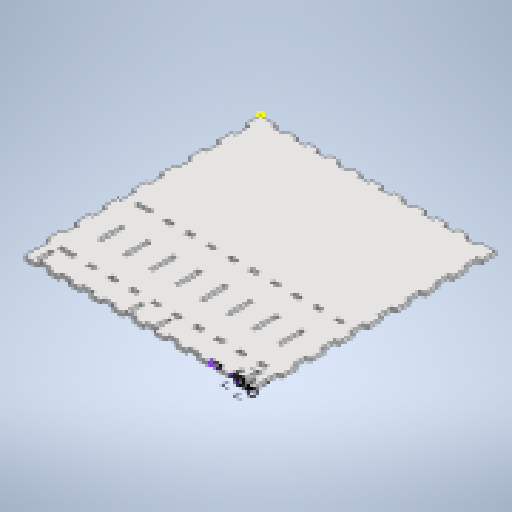
# Autodesk Inventor part: Bottom
Saved by Autodesk Inventor 2023 (Build 270158000, 158)
## iProperties
Created: 2023-08-30
Part Number: Bottom
Material: Generic
Document SubType Name: Modeling
Designer: Nathann
Density: 1 g/cm^3
Appearance: Default
Author: Nathann
Autodesk Inventor part; units mm, degrees
ref_plane "YZ Plane" through (0, 0, 0) normal (1, 0, 0) x (0, 1, 0)
ref_plane "XZ Plane" through (0, 0, 0) normal (0, 1, 0) x (-1, 0, 0)
ref_plane "XY Plane" through (0, 0, 0) normal (0, 0, 1) x (1, 0, 0)
sketch "Sketch1" plane through (0, 0, 0) normal (0, 1, 0) x (-1, 0, 0)
  line L0 (0, 0) -> (-330, 0)
  line L1 (-330, 0) -> (-330, 330)
  line L2 (-330, 330) -> (0, 330)
  line L3 (0, 330) -> (0, 0)
  dimension "d0" = 330
  dimension "d1" = 330
  constraints: 8 end point, 2 parallel, 1 horizontal, 1 perpendicular
  measures "d0" distance of L2.end L0.start
  measures "d1" distance of L1.end L2.end
extrude "Extrusion1" add sketch "Sketch1" along normal blind 5
sketch "Sketch4" plane through (0, 0, 0) normal (0, -1, 0) x (1, 0, 0)
  line L0 (325, 325) -> (307.5, 325) projected
  line L1 (325, 330) -> (325, 300) projected
  line L2 (307.5, 325) -> (307.5, 330) projected
  line L3 (0, 330) -> (330, 330) projected
  line L4 (297.5, 325) -> (297.5, 330)
  line L5 (277.5, 325) -> (277.5, 330) projected
  line L6 (292.5, 325) -> (277.5, 325) projected
  line L7 (292.5, 330) -> (292.5, 325) projected
  line L8 (262.5, 330) -> (262.5, 325) projected
  line L9 (262.5, 325) -> (247.5, 325) projected
  line L10 (247.5, 325) -> (247.5, 330) projected
  line L11 (232.5, 330) -> (232.5, 325) projected
  line L12 (232.5, 325) -> (217.5, 325) projected
  line L13 (217.5, 325) -> (217.5, 330) projected
  line L14 (202.5, 330) -> (202.5, 325) projected
  line L15 (202.5, 325) -> (187.5, 325) projected
  line L16 (187.5, 325) -> (187.5, 330) projected
  line L17 (172.5, 330) -> (172.5, 325) projected
  line L18 (172.5, 325) -> (157.5, 325) projected
  line L19 (157.5, 325) -> (157.5, 330) projected
  line L20 (142.5, 325) -> (127.5, 325) projected
  line L21 (142.5, 330) -> (142.5, 325) projected
  line L22 (127.5, 325) -> (127.5, 330) projected
  line L23 (112.5, 330) -> (112.5, 325) projected
  line L24 (112.5, 325) -> (97.5, 325) projected
  line L25 (97.5, 325) -> (97.5, 330) projected
  line L26 (82.5, 325) -> (67.5, 325) projected
  line L27 (82.5, 330) -> (82.5, 325) projected
  line L28 (67.5, 325) -> (67.5, 330) projected
  line L29 (52.5, 325) -> (37.5, 325) projected
  line L30 (52.5, 330) -> (52.5, 325) projected
  line L31 (37.5, 325) -> (37.5, 330) projected
  line L32 (22.5, 325) -> (5, 325) projected
  line L33 (22.5, 330) -> (22.5, 325) projected
  line L34 (5, 330) -> (5, 300) projected
  line L35 (292.5, 325) -> (307.5, 325) projected
  line L36 (262.5, 325) -> (277.5, 325) projected
  line L37 (232.5, 325) -> (247.5, 325) projected
  line L38 (202.5, 325) -> (217.5, 325) projected
  line L39 (172.5, 325) -> (187.5, 325) projected
  line L40 (142.5, 325) -> (157.5, 325) projected
  line L41 (112.5, 325) -> (127.5, 325) projected
  line L42 (82.5, 325) -> (97.5, 325) projected
  line L43 (52.5, 325) -> (67.5, 325) projected
  line L44 (22.5, 325) -> (37.5, 325) projected
  line L45 (0, 300) -> (5, 300) projected
  line L46 (5, 300) -> (5, 280) projected
  line L47 (0, 330) -> (0, 300) projected
  line L48 (0, 0) -> (0, 330) projected
  line L49 (5, 280) -> (0, 280) projected
  line L50 (5, 280) -> (5, 260) projected
  line L51 (0, 260) -> (5, 260) projected
  line L52 (5, 260) -> (5, 240) projected
  line L53 (5, 240) -> (0, 240) projected
  line L54 (5, 240) -> (0, 240) projected
  line L55 (0, 240) -> (0, 220) projected
  line L56 (0, 220) -> (5, 220) projected
  line L57 (5, 240) -> (5, 220) projected
  line L58 (5, 220) -> (5, 200) projected
  line L59 (5, 200) -> (0, 200) projected
  line L60 (5, 200) -> (5, 180) projected
  line L61 (0, 180) -> (5, 180) projected
  line L62 (5, 180) -> (5, 160) projected
  line L63 (5, 160) -> (0, 160) projected
  line L64 (5, 160) -> (5, 140) projected
  line L65 (0, 140) -> (5, 140) projected
  line L66 (5, 140) -> (5, 120) projected
  line L67 (5, 120) -> (0, 120) projected
  line L68 (5, 120) -> (5, 100) projected
  line L69 (0, 100) -> (5, 100) projected
  line L70 (5, 100) -> (5, 80) projected
  line L71 (5, 80) -> (0, 80) projected
  line L72 (5, 80) -> (5, 60) projected
  line L73 (0, 60) -> (5, 60) projected
  line L74 (5, 60) -> (5, 40) projected
  line L75 (5, 40) -> (0, 40) projected
  line L76 (5, 40) -> (5, 20) projected
  line L77 (0, 20) -> (5, 20) projected
  line L78 (5, 20) -> (5, 0) projected
  line L79 (330, 0) -> (0, 0) projected
  line L80 (5, 5) -> (22.5, 5) projected
  line L81 (22.5, 5) -> (22.5, 0) projected
  line L82 (37.5, 0) -> (37.5, 5) projected
  line L83 (22.5, 5) -> (37.5, 5) projected
  line L84 (45, 0) -> (45, 5) projected
  line L85 (37.5, 5) -> (52.5, 5) projected
  line L86 (52.5, 5) -> (52.5, 0) projected
  line L87 (52.5, 5) -> (67.5, 5) projected
  line L88 (67.5, 0) -> (67.5, 5) projected
  line L89 (67.5, 5) -> (82.5, 5) projected
  line L90 (82.5, 5) -> (82.5, 0) projected
  line L91 (82.5, 5) -> (97.5, 5) projected
  line L92 (97.5, 0) -> (97.5, 5) projected
  line L93 (112.5, 5) -> (112.5, 0) projected
  line L94 (97.5, 5) -> (112.5, 5) projected
  line L95 (112.5, 5) -> (127.5, 5) projected
  line L96 (127.5, 0) -> (127.5, 5) projected
  line L97 (127.5, 5) -> (142.5, 5) projected
  line L98 (142.5, 5) -> (142.5, 0) projected
  line L99 (142.5, 5) -> (157.5, 5) projected
  line L100 (157.5, 0) -> (157.5, 5) projected
  line L101 (157.5, 5) -> (172.5, 5) projected
  line L102 (172.5, 5) -> (172.5, 0) projected
  line L103 (172.5, 5) -> (187.5, 5) projected
  line L104 (187.5, 0) -> (187.5, 5) projected
  line L105 (187.5, 5) -> (202.5, 5) projected
  line L106 (202.5, 5) -> (202.5, 0) projected
  line L107 (202.5, 5) -> (217.5, 5) projected
  line L108 (217.5, 0) -> (217.5, 5) projected
  line L109 (217.5, 5) -> (232.5, 5) projected
  line L110 (232.5, 5) -> (232.5, 0) projected
  line L111 (232.5, 5) -> (247.5, 5) projected
  line L112 (247.5, 0) -> (247.5, 5) projected
  line L113 (247.5, 5) -> (262.5, 5) projected
  line L114 (262.5, 5) -> (262.5, 0) projected
  line L115 (262.5, 5) -> (277.5, 5) projected
  line L116 (277.5, 0) -> (277.5, 5) projected
  line L117 (277.5, 5) -> (292.5, 5) projected
  line L118 (292.5, 5) -> (292.5, 0) projected
  line L119 (292.5, 5) -> (307.5, 5) projected
  line L120 (307.5, 0) -> (307.5, 5) projected
  line L121 (307.5, 5) -> (325, 5) projected
  line L122 (325, 0) -> (325, 5) projected
  line L123 (325, 5) -> (330, 5) projected
  line L124 (325, 0) -> (325, 20) projected
  line L125 (325, 40) -> (325, 20) projected
  line L126 (325, 20) -> (330, 20) projected
  line L127 (325, 20) -> (330, 20) projected
  line L128 (330, 40) -> (330, 20) projected
  line L129 (330, 40) -> (325, 40) projected
  line L130 (325, 40) -> (325, 20) projected
  line L131 (325, 40) -> (325, 60) projected
  line L132 (325, 60) -> (330, 60) projected
  line L133 (330, 80) -> (325, 80) projected
  line L134 (325, 80) -> (325, 60) projected
  line L135 (325, 80) -> (325, 100) projected
  line L136 (325, 100) -> (330, 100) projected
  line L137 (325, 120) -> (325, 100) projected
  line L138 (330, 120) -> (325, 120) projected
  line L139 (325, 120) -> (325, 140) projected
  line L140 (325, 140) -> (330, 140) projected
  line L141 (325, 140) -> (330, 140) projected
  line L142 (330, 160) -> (330, 140) projected
  line L143 (330, 160) -> (325, 160) projected
  line L144 (325, 160) -> (325, 140) projected
  line L145 (325, 160) -> (325, 180) projected
  line L146 (325, 180) -> (330, 180) projected
  line L147 (330, 330) -> (330, 0) projected
  line L148 (330, 200) -> (325, 200) projected
  line L149 (325, 200) -> (325, 180) projected
  line L150 (325, 180) -> (330, 180) projected
  line L151 (330, 200) -> (330, 180) projected
  line L152 (325, 220) -> (330, 220) projected
  line L153 (325, 200) -> (325, 220) projected
  line L154 (325, 240) -> (325, 220) projected
  line L155 (330, 240) -> (325, 240) projected
  line L156 (325, 240) -> (325, 260) projected
  line L157 (325, 260) -> (330, 260) projected
  line L158 (325, 280) -> (325, 260) projected
  line L159 (330, 280) -> (325, 280) projected
  line L160 (325, 280) -> (325, 300) projected
  line L161 (325, 300) -> (330, 300) projected
  line L162 (330, 325) -> (325, 325) projected
  line L163 (293.8889, 264) -> (288.8889, 264) projected
  line L164 (257.7778, 299) -> (257.7778, 264) projected
  line L165 (252.7778, 264) -> (252.7778, 299) projected
  line L166 (257.7778, 264) -> (252.7778, 264) projected
  line L167 (221.6667, 299) -> (221.6667, 264) projected
  line L168 (216.6667, 264) -> (216.6667, 299) projected
  line L169 (221.6667, 264) -> (216.6667, 264) projected
  line L170 (221.6667, 264) -> (221.6667, 231) projected
  line L171 (216.6667, 231) -> (216.6667, 264) projected
  line L172 (216.6667, 231) -> (221.6667, 231) projected
  line L173 (257.7778, 264) -> (257.7778, 231) projected
  line L174 (257.7778, 264) -> (252.7778, 264) projected
  line L175 (252.7778, 231) -> (252.7778, 264) projected
  line L176 (252.7778, 231) -> (257.7778, 231) projected
  line L177 (257.7778, 264) -> (257.7778, 231) projected
  line L178 (293.8889, 264) -> (288.8889, 264) projected
  line L179 (288.8889, 231) -> (288.8889, 264) projected
  line L180 (288.8889, 231) -> (293.8889, 231) projected
  line L181 (293.8889, 264) -> (293.8889, 231) projected
  line L182 (185.5556, 264) -> (180.5556, 264) projected
  line L183 (180.5556, 231) -> (180.5556, 264) projected
  line L184 (180.5556, 231) -> (185.5556, 231) projected
  line L185 (185.5556, 264) -> (185.5556, 231) projected
  line L186 (185.5556, 299) -> (185.5556, 264) projected
  line L187 (180.5556, 264) -> (180.5556, 299) projected
  line L188 (149.4444, 264) -> (144.4444, 264) projected
  line L189 (144.4444, 231) -> (144.4444, 264) projected
  line L190 (144.4444, 231) -> (149.4444, 231) projected
  line L191 (149.4444, 264) -> (149.4444, 231) projected
  line L192 (113.3333, 264) -> (108.3333, 264) projected
  line L193 (108.3333, 231) -> (108.3333, 264) projected
  line L194 (108.3333, 231) -> (113.3333, 231) projected
  line L195 (113.3333, 264) -> (113.3333, 231) projected
  line L196 (77.2222, 264) -> (72.2222, 264) projected
  line L197 (72.2222, 231) -> (72.2222, 264) projected
  line L198 (72.2222, 231) -> (77.2222, 231) projected
  line L199 (77.2222, 264) -> (77.2222, 231) projected
  line L200 (41.1111, 264) -> (36.1111, 264) projected
  line L201 (36.1111, 231) -> (36.1111, 264) projected
  line L202 (36.1111, 231) -> (41.1111, 231) projected
  line L203 (41.1111, 264) -> (41.1111, 231) projected
  line L204 (20, 196) -> (40, 196) projected
  line L205 (40, 191) -> (40, 196) projected
  line L206 (20, 196) -> (40, 196) projected
  line L207 (20, 196) -> (20, 191) projected
  line L208 (20, 191) -> (40, 191) projected
  line L209 (60, 196) -> (60, 191) projected
  line L210 (60, 191) -> (70, 191) projected
  line L211 (70, 191) -> (70, 196) projected
  line L212 (60, 196) -> (70, 196) projected
  line L213 (100, 191) -> (100, 196) projected
  line L214 (90, 196) -> (100, 196) projected
  line L215 (90, 196) -> (90, 191) projected
  line L216 (90, 191) -> (100, 191) projected
  line L217 (120, 196) -> (120, 191) projected
  line L218 (120, 191) -> (130, 191) projected
  line L219 (130, 191) -> (130, 196) projected
  line L220 (120, 196) -> (130, 196) projected
  line L221 (160, 191) -> (160, 196) projected
  line L222 (150, 196) -> (160, 196) projected
  line L223 (150, 196) -> (150, 191) projected
  line L224 (150, 191) -> (160, 191) projected
  line L225 (180, 196) -> (180, 191) projected
  line L226 (180, 191) -> (190, 191) projected
  line L227 (190, 191) -> (190, 196) projected
  line L228 (180, 196) -> (190, 196) projected
  line L229 (216.6667, 191) -> (216.6667, 196) projected
  line L230 (210, 196) -> (210, 191) projected
  line L231 (210, 191) -> (220, 191) projected
  line L232 (220, 191) -> (220, 196) projected
  line L233 (210, 196) -> (220, 196) projected
  line L234 (250, 191) -> (250, 196) projected
  line L235 (240, 196) -> (250, 196) projected
  line L236 (240, 196) -> (240, 191) projected
  line L237 (240, 191) -> (250, 191) projected
  line L238 (280, 191) -> (280, 196) projected
  line L239 (270, 196) -> (280, 196) projected
  line L240 (270, 196) -> (270, 191) projected
  line L241 (270, 191) -> (280, 191) projected
  line L242 (300, 196) -> (300, 191) projected
  line L243 (300, 191) -> (310, 191) projected
  line L244 (310, 191) -> (310, 196) projected
  line L245 (300, 196) -> (310, 196) projected
  line L246 (300, 191) -> (280, 191) projected
  point P0 (181.5, 325)
  constraints: 2 end point, 1 vertical, 7 other
extrude "Extrusion2" cut sketch "Sketch4" against normal blind 10 contours L162 L147 L161 L1 | L1 L3 L147 L162 | L35 L4 L3 L2 | L35 L7 L3 L4 | L159 L147 L157 L158 | L36 L8 L3 L5 | L155 L147 L152 L154 | L37 L11 L3 L10 | L148 L147 L146 L149 | L38 L14 L3 L13 | L143 L142 L140 L144 | L39 L17 L3 L16 | L138 L147 L136 L137 | L40 L21 L3 L19 | L133 L147 L132 L134 | L41 L23 L3 L22 | L129 L128 L126 L125 | L42 L27 L3 L25 | L120 L79 L118 L119 | L43 L30 L3 L28 | L116 L79 L114 L115 | L44 L33 L3 L31 | L112 L79 L110 L111 | L34 L45 L47 L3 | L108 L79 L106 L107 | L50 L51 L48 L49 | L104 L79 L102 L103 | L57 L56 L48 L53 | L100 L79 L98 L99 | L60 L61 L48 L59 | L96 L79 L93 L95 | L64 L65 L48 L63 | L92 L79 L90 L91 | L68 L69 L48 L67 | L88 L79 L86 L87 | L72 L73 L48 L71 | L76 L77 L48 L75 | L82 L79 L81 L83 | L181 L180 L179 L163 | L173 L176 L175 L166 | L170 L172 L171 L169 | L185 L184 L183 L182 | L191 L190 L189 L188 | L195 L194 L193 L192 | L199 L198 L197 L196 | L203 L202 L201 L200 | L204 L205 L208 L207 | L212 L211 L210 L209 | L216 L215 L214 L213 | L220 L219 L218 L217 | L224 L223 L222 L221 | L228 L227 L226 L225 | L231 L230 L233 L229 | L229 L233 L232 L231 | L237 L236 L235 L234 | L241 L240 L239 L238 | L242 L245 L244 L243
sketch "Sketch5" plane through (0, 0, 0) normal (0, -1, 0) x (1, 0, 0)
  line L0 (325, 304) -> (5, 304) projected
  line L1 (5, 299) -> (325, 299) projected
  line L2 (313.5, 304) -> (313.5, 325) projected
  line L3 (308.5, 304) -> (313.5, 304) projected
  line L4 (308.5, 325) -> (308.5, 304) projected
  line L5 (313.5, 325) -> (308.5, 325) projected
  line L6 (186.5, 304) -> (186.5, 325) projected
  line L7 (181.5, 304) -> (186.5, 304) projected
  line L8 (181.5, 325) -> (181.5, 304) projected
  line L9 (186.5, 325) -> (181.5, 325) projected
  line L10 (148.5, 304) -> (148.5, 325) projected
  line L11 (143.5, 304) -> (148.5, 304) projected
  line L12 (143.5, 325) -> (143.5, 304) projected
  line L13 (148.5, 325) -> (143.5, 325) projected
  line L14 (21.5, 304) -> (21.5, 325) projected
  line L15 (16.5, 304) -> (21.5, 304) projected
  line L16 (16.5, 325) -> (16.5, 304) projected
  line L17 (21.5, 325) -> (16.5, 325) projected
  line L18 (143.5, 310) -> (148.5, 310) projected
  line L19 (181.5, 310) -> (186.5, 310) projected
  line L20 (16.5, 310) -> (21.5, 310) projected
  line L21 (308.5, 310) -> (313.5, 310) projected
  line L22 (310, 299) -> (310, 304) projected
  line L23 (300, 304) -> (300, 299) projected
  line L24 (293.8889, 304) -> (293.8889, 299) projected
  line L25 (288.8889, 304) -> (288.8889, 299) projected
  line L26 (270, 304) -> (270, 299) projected
  line L27 (270, 299) -> (280, 299) projected
  line L28 (280, 299) -> (280, 304) projected
  line L29 (270, 304) -> (280, 304) projected
  line L30 (257.7778, 304) -> (257.7778, 299) projected
  line L31 (250, 299) -> (250, 304) projected
  line L32 (240, 304) -> (250, 304) projected
  line L33 (240, 304) -> (240, 299) projected
  line L34 (240, 299) -> (250, 299) projected
  line L35 (210, 304) -> (210, 299) projected
  line L36 (210, 299) -> (220, 299) projected
  line L37 (220, 299) -> (220, 304) projected
  line L38 (210, 304) -> (220, 304) projected
  line L39 (190, 299) -> (190, 304) projected
  line L40 (180, 304) -> (190, 304) projected
  line L41 (180, 304) -> (180, 299) projected
  line L42 (180, 299) -> (190, 299) projected
  line L43 (120, 304) -> (120, 299) projected
  line L44 (120, 299) -> (130, 299) projected
  line L45 (130, 299) -> (130, 304) projected
  line L46 (120, 304) -> (130, 304) projected
  line L47 (20, 304) -> (20, 299) projected
  line L48 (20, 299) -> (40, 299) projected
  line L49 (40, 299) -> (40, 304) projected
  line L50 (20, 304) -> (40, 304) projected
  line L51 (60, 304) -> (60, 299) projected
  line L52 (60, 299) -> (70, 299) projected
  line L53 (70, 299) -> (70, 304) projected
  line L54 (60, 304) -> (70, 304) projected
  line L55 (100, 299) -> (100, 304) projected
  line L56 (90, 304) -> (100, 304) projected
  line L57 (90, 304) -> (90, 299) projected
  line L58 (90, 299) -> (100, 299) projected
  line L59 (108.3333, 304) -> (108.3333, 299) projected
  line L60 (113.3333, 304) -> (113.3333, 299) projected
  line L61 (144.4444, 304) -> (144.4444, 299) projected
  line L62 (150, 304) -> (150, 299) projected
  line L63 (149.4444, 304) -> (149.4444, 299) projected
  line L64 (160, 299) -> (160, 304) projected
  point P0 (0, 0)
  constraints: 2 other
extrude "Extrusion3" cut sketch "Sketch5" against normal blind 10 contours L22 L1 L23 L0 | L21 L4 L5 L2 | L28 L1 L26 L0 | L31 L1 L33 L0 | L37 L1 L35 L0 | L39 L1 L41 L0 | L19 L8 L9 L6 | L1 L62 L0 L64 | L1 L43 L0 L45 | L18 L12 L13 L10 | L1 L57 L0 L55 | L1 L51 L0 L53 | L1 L47 L0 L49 | L20 L16 L17 L14
sketch "Sketch6" plane through (0, 0, 0) normal (0, -1, 0) x (1, 0, 0)
  line L0 (325, 300) -> (325, 330) projected
  line L1 (325, 330) -> (307.5, 330)
  line L2 (307.5, 330) -> (307.5, 336)
  line L3 (307.5, 336) -> (325, 336)
  line L4 (325, 336) -> (325, 330)
  line L5 (307.5, 325) -> (292.5, 325) projected
  line L6 (307.5, 325) -> (292.5, 325)
  line L7 (292.5, 325) -> (292.5, 331)
  line L8 (292.5, 331) -> (307.5, 331)
  line L9 (307.5, 331) -> (307.5, 325)
  line L10 (277.5, 330) -> (292.5, 330) projected
  line L11 (292.5, 330) -> (277.5, 330)
  line L12 (277.5, 330) -> (277.5, 336)
  line L13 (277.5, 336) -> (292.5, 336)
  line L14 (292.5, 336) -> (292.5, 330)
  line L15 (277.5, 330) -> (277.5, 325) projected
  line L16 (277.5, 325) -> (262.5, 325)
  line L17 (262.5, 325) -> (262.5, 331)
  line L18 (262.5, 331) -> (277.5, 331)
  line L19 (277.5, 331) -> (277.5, 325)
  line L20 (262.5, 325) -> (262.5, 330) projected
  line L21 (262.5, 330) -> (247.5, 330)
  line L22 (247.5, 330) -> (247.5, 336)
  line L23 (247.5, 336) -> (262.5, 336)
  line L24 (262.5, 336) -> (262.5, 330)
  line L25 (247.5, 330) -> (247.5, 325) projected
  line L26 (247.5, 325) -> (232.5, 325)
  line L27 (232.5, 325) -> (232.5, 331)
  line L28 (232.5, 331) -> (247.5, 331)
  line L29 (247.5, 331) -> (247.5, 325)
  line L30 (217.5, 330) -> (232.5, 330) projected
  line L31 (232.5, 330) -> (217.5, 330)
  line L32 (217.5, 330) -> (217.5, 336)
  line L33 (217.5, 336) -> (232.5, 336)
  line L34 (232.5, 336) -> (232.5, 330)
  line L35 (217.5, 325) -> (202.5, 325) projected
  line L36 (217.5, 325) -> (202.5, 325)
  line L37 (202.5, 325) -> (202.5, 331)
  line L38 (202.5, 331) -> (217.5, 331)
  line L39 (217.5, 331) -> (217.5, 325)
  line L40 (202.5, 325) -> (202.5, 330) projected
  line L41 (202.5, 330) -> (187.5, 330)
  line L42 (187.5, 330) -> (187.5, 336)
  line L43 (187.5, 336) -> (202.5, 336)
  line L44 (202.5, 336) -> (202.5, 330)
  line L45 (187.5, 330) -> (187.5, 325) projected
  line L46 (187.5, 325) -> (172.5, 325)
  line L47 (172.5, 325) -> (172.5, 331)
  line L48 (172.5, 331) -> (187.5, 331)
  line L49 (187.5, 331) -> (187.5, 325)
  line L50 (172.5, 325) -> (172.5, 330) projected
  line L51 (172.5, 330) -> (157.5, 330)
  line L52 (157.5, 330) -> (157.5, 336)
  line L53 (157.5, 336) -> (172.5, 336)
  line L54 (172.5, 336) -> (172.5, 330)
  line L55 (148.5, 325) -> (157.5, 325) projected
  line L56 (157.5, 325) -> (142.5, 325)
  line L57 (142.5, 325) -> (142.5, 331)
  line L58 (142.5, 331) -> (157.5, 331)
  line L59 (157.5, 331) -> (157.5, 325)
  line L60 (127.5, 330) -> (142.5, 330) projected
  line L61 (142.5, 330) -> (127.5, 330)
  line L62 (127.5, 330) -> (127.5, 336)
  line L63 (127.5, 336) -> (142.5, 336)
  line L64 (142.5, 336) -> (142.5, 330)
  line L65 (127.5, 330) -> (127.5, 325) projected
  line L66 (127.5, 325) -> (112.5, 325)
  line L67 (112.5, 325) -> (112.5, 331)
  line L68 (112.5, 331) -> (127.5, 331)
  line L69 (127.5, 331) -> (127.5, 325)
  line L70 (97.5, 330) -> (112.5, 330) projected
  line L71 (112.5, 330) -> (97.5, 330)
  line L72 (97.5, 330) -> (97.5, 336)
  line L73 (97.5, 336) -> (112.5, 336)
  line L74 (112.5, 336) -> (112.5, 330)
  line L75 (97.5, 325) -> (82.5, 325) projected
  line L76 (97.5, 325) -> (82.5, 325)
  line L77 (82.5, 325) -> (82.5, 331)
  line L78 (82.5, 331) -> (97.5, 331)
  line L79 (97.5, 331) -> (97.5, 325)
  line L80 (82.5, 325) -> (82.5, 330) projected
  line L81 (82.5, 330) -> (67.5, 330)
  line L82 (67.5, 330) -> (67.5, 336)
  line L83 (67.5, 336) -> (82.5, 336)
  line L84 (82.5, 336) -> (82.5, 330)
  line L85 (67.5, 325) -> (52.5, 325) projected
  line L86 (67.5, 325) -> (52.5, 325)
  line L87 (52.5, 325) -> (52.5, 331)
  line L88 (52.5, 331) -> (67.5, 331)
  line L89 (67.5, 331) -> (67.5, 325)
  line L90 (52.5, 325) -> (52.5, 330) projected
  line L91 (52.5, 330) -> (37.5, 330)
  line L92 (37.5, 330) -> (37.5, 336)
  line L93 (37.5, 336) -> (52.5, 336)
  line L94 (52.5, 336) -> (52.5, 330)
  line L95 (37.5, 330) -> (37.5, 325) projected
  line L96 (37.5, 325) -> (22.5, 325)
  line L97 (22.5, 325) -> (22.5, 331)
  line L98 (22.5, 331) -> (37.5, 331)
  line L99 (37.5, 331) -> (37.5, 325)
  line L100 (5, 330) -> (22.5, 330) projected
  line L101 (22.5, 330) -> (5, 330)
  line L102 (5, 330) -> (5, 336)
  line L103 (5, 336) -> (22.5, 336)
  line L104 (22.5, 336) -> (22.5, 330)
  point P0 (0, 0)
  dimension "d8" = 6
  dimension "d9" = 6
  constraints: 168 end point, 42 parallel, 21 horizontal, 21 perpendicular, 17 point on line
  measures "d8" distance of L1.end L2.end
  measures "d9" distance between parallel lines of L5 L8
extrude "Extrusion4" add sketch "Sketch6" against normal blind 5
sketch "Sketch7" plane through (0, 0, 0) normal (0, -1, 0) x (1, 0, 0)
  line L0 (313.5, 310) -> (313.5, 325) projected
  line L1 (313.5, 325) -> (308.5, 325)
  line L2 (308.5, 325) -> (308.5, 331)
  line L3 (308.5, 331) -> (313.5, 331)
  line L4 (313.5, 331) -> (313.5, 325)
  line L5 (186.5, 325) -> (181.5, 325) projected
  line L6 (186.5, 325) -> (181.5, 325)
  line L7 (181.5, 325) -> (181.5, 331)
  line L8 (181.5, 331) -> (186.5, 331)
  line L9 (186.5, 331) -> (186.5, 325)
  line L10 (143.5, 325) -> (148.5, 325) projected
  line L11 (148.5, 325) -> (143.5, 325)
  line L12 (143.5, 325) -> (143.5, 331)
  line L13 (143.5, 331) -> (148.5, 331)
  line L14 (148.5, 331) -> (148.5, 325)
  line L15 (16.5, 325) -> (21.5, 325) projected
  line L16 (21.5, 325) -> (16.5, 325)
  line L17 (16.5, 325) -> (16.5, 331)
  line L18 (16.5, 331) -> (21.5, 331)
  line L19 (21.5, 331) -> (21.5, 325)
  point P0 (0, 0)
  dimension "d12" = 6
  dimension "d15" = 6
  dimension "d16" = 6
  dimension "d17" = 6
  constraints: 32 end point, 8 parallel, 4 horizontal, 4 perpendicular, 2 point on line
  measures "d12" distance between parallel lines of L1 L3
  measures "d15" distance of L8.end L5.start
  measures "d16" distance of L13.end L10.end
  measures "d17" distance of L18.end L15.end
extrude "Extrusion5" cut sketch "Sketch7" against normal blind 5
sketch "Sketch8" plane through (0, 0, 0) normal (0, -1, 0) x (1, 0, 0)
  line L0 (313.5, 310) -> (313.5, 331) projected
  line L1 (16.5, 331) -> (16.5, 310) projected
  line L2 (313.5, 310) -> (16.5, 310)
  line L3 (16.5, 310) -> (16.5, 311)
  line L4 (16.5, 311) -> (313.5, 311)
  line L5 (313.5, 311) -> (313.5, 310)
  point P0 (0, 0)
  dimension "d18" = 1
  constraints: 8 end point, 2 parallel, 1 horizontal, 1 perpendicular, 1 point on line
  measures "d18" distance between parallel lines of L2 L4
extrude "Extrusion6" add sketch "Sketch8" against normal blind 5
sketch "Sketch9" plane through (0, 5, 0) normal (0, 1, 0) x (1, 0, 0)
  line L0 (325, -336) -> (307.5, -336) projected
  line L1 (325, -336) -> (307.5, -336)
  line L2 (307.5, -336) -> (307.5, -342)
  line L3 (307.5, -342) -> (325, -342)
  line L4 (325, -342) -> (325, -336)
  line L5 (307.5, -336) -> (307.5, -331) projected
  line L6 (307.5, -331) -> (292.5, -331)
  line L7 (292.5, -331) -> (292.5, -337)
  line L8 (292.5, -337) -> (307.5, -337)
  line L9 (307.5, -337) -> (307.5, -331)
  line L10 (277.5, -331) -> (262.5, -331) projected
  line L11 (277.5, -331) -> (262.5, -331)
  line L12 (262.5, -331) -> (262.5, -337.5909)
  line L13 (262.5, -337.5909) -> (277.5, -337.5909)
  line L14 (277.5, -337.5909) -> (277.5, -331)
  point P0 (0, 0)
  dimension "d21" = 6
  dimension "d22" = 6
  constraints: 24 end point, 6 parallel, 3 horizontal, 3 perpendicular
  measures "d21" distance of L3.end L0.start
  measures "d22" distance between parallel lines of L8 L6
sketch "Sketch10" plane through (0, 0, 0) normal (0, -1, 0) x (1, 0, 0)
  point P0 (0, 0)
body "Solid1"
